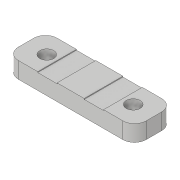
# Autodesk Inventor part: 8 peristaltic pump clamp 0.2mm
Saved by Autodesk Inventor 2020 (Build 240168000, 168)
## iProperties
Created: 2018-08-21
Part Number: 8 peristaltic pump clamp 0.2mm
Material: Generic
Document SubType Name: Modeling
Designer: mrbeh
Density: 1 g/cm^3
Appearance: Default
Author: mrbeh
Autodesk Inventor part; units mm, degrees
ref_plane "YZ Plane" through (0, 0, 0) normal (1, 0, 0) x (0, 1, 0)
ref_plane "XZ Plane" through (0, 0, 0) normal (0, 1, 0) x (-1, 0, 0)
sketch "Sketch1" plane through (0, 0, 0) normal (0, 1, 0) x (-1, 0, 0)
  line L0 (0, 0) -> (33, 0)
  line L1 (33, 0) -> (33, -10)
  line L2 (33, -10) -> (0, -10)
  line L3 (0, -10) -> (0, 0)
  dimension "d0" = 33
  dimension "d1" = 10
  constraints: 8 end point, 2 parallel, 1 horizontal, 1 perpendicular
  measures "d0" distance of L1.end L2.end
  measures "d1" distance of L0.end L1.end
extrude "Extrusion1" add sketch "Sketch1" along normal blind 4
sketch "Sketch2" plane through (0, 4, 0) normal (0, 1, 0) x (1, 0, 0)
  circle A0 centre (-5.343, 5) radius 1.8
  point P0 (0, 0)
  dimension "d9" = 3.6
  constraints: 1 centre point
  measures "d9" diameter of A0
extrude "Extrusion2" cut sketch "Sketch2" against normal blind 4
ref_plane "Work Plane1" through (-16.5, 0, 0) normal (1, 0, 0) x (0, 0, -1)
mirror "Mirror1" about plane through (-16.5, 0, 0) normal (1, 0, 0) of "Extrusion2"
fillet "Fillet1" radius 3 4 edges at (-33, 2, 0) (-33, 2, -10) (0, 2, 0) (0, 2, -10)
sketch "Sketch3" plane through (0, 4, 0) normal (0, 1, 0) x (1, 0, 0)
  line L0 (-30, 0) -> (-3, 0) projected
  line L1 (-30, 10) -> (-3, 10) projected
  line L2 (-20, 0) -> (-13, 0)
  line L3 (-13, 0) -> (-13, 10)
  line L4 (-13, 10) -> (-20, 10)
  line L5 (-20, 10) -> (-20, 0)
  point P0 (0, 0)
  dimension "d10" = 7
  dimension "d11" = 10
  constraints: 8 end point, 2 parallel, 1 horizontal, 1 perpendicular, 1 point on line
  measures "d10" distance of L4.end L3.end
  measures "d11" distance of L3.end L2.end
extrude "Extrusion3" add sketch "Sketch3" along normal blind 0.2
sketch "Sketch4" plane through (0, 4, 0) normal (0, 1, 0) x (1, 0, 0)
  line L0 (-3, 0) -> (-8, 0)
  line L1 (-8, 0) -> (-8, 10)
  line L2 (-8, 10) -> (-3, 10)
  line L3 (0, 7) -> (0, 3)
  arc A0 (-3, 0) -> (0, 3) centre (-3, 3) ccw
  arc A1 (0, 7) -> (-3, 10) centre (-3, 7) ccw
  circle A2 centre (-5.343, 5) radius 1.8 projected
  circle A3 centre (-5.343, 5) radius 1.8
  point P0 (0, 0)
  point P1 (0, 10)
  dimension "d14" = 8
  dimension "d15" = 10
  dimension "d16" = 3
  constraints: 8 end point, 4 point on circle, 4 point on line, 4 tangent, 3 centre point, 2 parallel, 1 coincident, 1 equal radius, 1 horizontal, 1 perpendicular
  measures "d14" distance of L1.end point (0, 10)
  measures "d15" distance of L0.end L1.end
  measures "d16" radius of A0
extrude "Extrusion4" add sketch "Sketch4" along normal blind 0.2
mirror "Mirror2" about plane through (-16.5, 0, 0) normal (1, 0, 0) of "Extrusion4"
sketch "Sketch5" plane through (0, 0, 0) normal (0, -1, 0) x (1, 0, 0)
  line L0 (-24.4942, -3.2042) -> (-8.1968, -3.2042) construction
  line L1 (-8.1968, -3.2042) -> (-8.1968, -6.8489) construction
  line L2 (-8.1968, -6.8489) -> (-24.4942, -6.8489) construction
  line L3 (-24.4942, -6.8489) -> (-24.4942, -3.2042) construction
  spline S0 degree 2 poles (-22.0607, -5.028) (-22.0607, -5.9696) (-22.6081, -6.8517) (-23.1782, -6.8517) knots 0 0 0 1 2 2 2
  spline S1 degree 2 poles (-23.1782, -6.8517) (-23.7568, -6.8517) (-24.2985, -5.9526) (-24.2985, -5.0308) knots 0 0 0 1 2 2 2
  spline S2 degree 2 poles (-24.2985, -5.0308) (-24.2985, -4.0835) (-23.7511, -3.2071) (-23.1782, -3.2071) knots 0 0 0 1 2 2 2
  spline S3 degree 2 poles (-23.1782, -3.2071) (-22.6024, -3.2071) (-22.0607, -4.1147) (-22.0607, -5.028) knots 0 0 0 1 2 2 2
  spline S4 degree 2 poles (-22.662, -6.0944) (-22.5939, -5.9214) (-22.5372, -5.3882) (-22.5372, -5.028) knots 0 0 0 1 2 2 2
  spline S5 degree 2 poles (-22.5372, -5.028) (-22.5372, -4.6678) (-22.5939, -4.1374) (-22.6648, -3.9587) knots 0 0 0 1 2 2 2
  spline S6 degree 2 poles (-22.6648, -3.9587) (-22.7357, -3.78) (-22.9825, -3.5957) (-23.1782, -3.5957) knots 0 0 0 1 2 2 2
  spline S7 degree 2 poles (-23.1782, -3.5957) (-23.3739, -3.5957) (-23.6263, -3.78) (-23.7, -3.9644) knots 0 0 0 1 2 2 2
  spline S8 degree 2 poles (-23.7, -3.9644) (-23.7709, -4.1431) (-23.822, -4.6876) (-23.822, -5.0308) knots 0 0 0 1 2 2 2
  spline S9 degree 2 poles (-23.822, -5.0308) (-23.822, -5.3995) (-23.7766, -5.8931) (-23.7029, -6.0859) knots 0 0 0 1 2 2 2
  spline S10 degree 2 poles (-23.7029, -6.0859) (-23.6348, -6.2675) (-23.3824, -6.4632) (-23.1782, -6.4632) knots 0 0 0 1 2 2 2
  spline S11 degree 2 poles (-23.1782, -6.4632) (-22.9853, -6.4632) (-22.7329, -6.2788) (-22.662, -6.0944) knots 0 0 0 1 2 2 2
  line L4 (-20.8609, -6.778) -> (-21.4225, -6.778)
  line L5 (-21.4225, -6.778) -> (-21.4225, -6.1086)
  line L6 (-21.4225, -6.1086) -> (-20.8609, -6.1086)
  line L7 (-20.8609, -6.1086) -> (-20.8609, -6.778)
  line L8 (-17.9962, -6.778) -> (-20.1547, -6.778)
  line L9 (-20.1547, -6.778) -> (-20.1547, -6.2816)
  spline S12 degree 2 poles (-20.1547, -6.2816) (-19.9221, -6.0632) (-19.508, -5.6576) (-19.3094, -5.4393) knots 0 0 0 1 2 2 2
  spline S13 degree 2 poles (-19.3094, -5.4393) (-18.9095, -4.9996) (-18.6174, -4.4721) (-18.6174, -4.1913) knots 0 0 0 1 2 2 2
  spline S14 degree 2 poles (-18.6174, -4.1913) (-18.6174, -4.0438) (-18.7081, -3.8226) (-18.7904, -3.7517) knots 0 0 0 1 2 2 2
  spline S15 degree 2 poles (-18.7904, -3.7517) (-18.8727, -3.6807) (-19.0882, -3.6098) (-19.2187, -3.6098) knots 0 0 0 1 2 2 2
  spline S16 degree 2 poles (-19.2187, -3.6098) (-19.3435, -3.6098) (-19.5987, -3.6722) (-19.715, -3.7205) knots 0 0 0 1 2 2 2
  spline S17 degree 2 poles (-19.715, -3.7205) (-19.8143, -3.7602) (-19.9987, -3.8736) (-20.0554, -3.9133) knots 0 0 0 1 2 2 2
  line L10 (-20.0554, -3.9133) -> (-20.0809, -3.9133)
  line L11 (-20.0809, -3.9133) -> (-20.0809, -3.4141)
  spline S18 degree 2 poles (-20.0809, -3.4141) (-19.9363, -3.3432) (-19.4172, -3.2042) (-19.1846, -3.2042) knots 0 0 0 1 2 2 2
  spline S19 degree 2 poles (-19.1846, -3.2042) (-18.694, -3.2042) (-18.1409, -3.7233) (-18.1409, -4.1658) knots 0 0 0 1 2 2 2
  spline S20 degree 2 poles (-18.1409, -4.1658) (-18.1409, -4.3728) (-18.2373, -4.7188) (-18.3224, -4.8663) knots 0 0 0 1 2 2 2
  spline S21 degree 2 poles (-18.3224, -4.8663) (-18.4075, -5.0195) (-18.6543, -5.3201) (-18.7904, -5.4648) knots 0 0 0 1 2 2 2
  spline S22 degree 2 poles (-18.7904, -5.4648) (-19.0116, -5.7059) (-19.5534, -6.2221) (-19.715, -6.3724) knots 0 0 0 1 2 2 2
  line L12 (-19.715, -6.3724) -> (-17.9962, -6.3724)
  line L13 (-17.9962, -6.3724) -> (-17.9962, -6.778)
  line L14 (-12.9816, -6.778) -> (-12.9816, -5.2577)
  spline S23 degree 2 poles (-12.9816, -5.2577) (-12.9816, -5.0762) (-13.01, -4.7671) (-13.0554, -4.682) knots 0 0 0 1 2 2 2
  spline S24 degree 2 poles (-13.0554, -4.682) (-13.1008, -4.5884) (-13.2738, -4.4976) (-13.4241, -4.4976) knots 0 0 0 1 2 2 2
  spline S25 degree 2 poles (-13.4241, -4.4976) (-13.5603, -4.4976) (-13.8722, -4.6649) (-14.0368, -4.8238) knots 0 0 0 1 2 2 2
  spline S26 degree 2 poles (-14.0368, -4.8238) (-14.0339, -4.8635) (-14.0282, -4.9741) (-14.0282, -5.0478) knots 0 0 0 1 2 2 2
  line L15 (-14.0282, -5.0478) -> (-14.0282, -6.778)
  line L16 (-14.0282, -6.778) -> (-14.4707, -6.778)
  line L17 (-14.4707, -6.778) -> (-14.4707, -5.2577)
  spline S27 degree 2 poles (-14.4707, -5.2577) (-14.4707, -5.0762) (-14.4991, -4.7671) (-14.5444, -4.682) knots 0 0 0 1 2 2 2
  spline S28 degree 2 poles (-14.5444, -4.682) (-14.5898, -4.5884) (-14.7628, -4.4976) (-14.9132, -4.4976) knots 0 0 0 1 2 2 2
  spline S29 degree 2 poles (-14.9132, -4.4976) (-15.055, -4.4976) (-15.3698, -4.6763) (-15.5173, -4.8153) knots 0 0 0 1 2 2 2
  line L18 (-15.5173, -4.8153) -> (-15.5173, -6.778)
  line L19 (-15.5173, -6.778) -> (-15.9598, -6.778)
  line L20 (-15.9598, -6.778) -> (-15.9598, -4.1516)
  line L21 (-15.9598, -4.1516) -> (-15.5173, -4.1516)
  line L22 (-15.5173, -4.1516) -> (-15.5173, -4.4409)
  spline S30 degree 2 poles (-15.5173, -4.4409) (-15.3443, -4.2679) (-15.0039, -4.0778) (-14.7997, -4.0778) knots 0 0 0 1 2 2 2
  spline S31 degree 2 poles (-14.7997, -4.0778) (-14.5671, -4.0778) (-14.2069, -4.2906) (-14.1133, -4.5316) knots 0 0 0 1 2 2 2
  spline S32 degree 2 poles (-14.1133, -4.5316) (-13.912, -4.3076) (-13.5319, -4.0778) (-13.3107, -4.0778) knots 0 0 0 1 2 2 2
  spline S33 degree 2 poles (-13.3107, -4.0778) (-13.1405, -4.0778) (-12.8625, -4.1828) (-12.7604, -4.3019) knots 0 0 0 1 2 2 2
  spline S34 degree 2 poles (-12.7604, -4.3019) (-12.6555, -4.421) (-12.5392, -4.7784) (-12.5392, -5.0478) knots 0 0 0 1 2 2 2
  line L23 (-12.5392, -5.0478) -> (-12.5392, -6.778)
  line L24 (-12.5392, -6.778) -> (-12.9816, -6.778)
  line L25 (-8.9399, -6.778) -> (-8.9399, -5.2577)
  spline S35 degree 2 poles (-8.9399, -5.2577) (-8.9399, -5.0762) (-8.9683, -4.7671) (-9.0137, -4.682) knots 0 0 0 1 2 2 2
  spline S36 degree 2 poles (-9.0137, -4.682) (-9.059, -4.5884) (-9.2321, -4.4976) (-9.3824, -4.4976) knots 0 0 0 1 2 2 2
  spline S37 degree 2 poles (-9.3824, -4.4976) (-9.5185, -4.4976) (-9.8305, -4.6649) (-9.995, -4.8238) knots 0 0 0 1 2 2 2
  spline S38 degree 2 poles (-9.995, -4.8238) (-9.9922, -4.8635) (-9.9865, -4.9741) (-9.9865, -5.0478) knots 0 0 0 1 2 2 2
  line L26 (-9.9865, -5.0478) -> (-9.9865, -6.778)
  line L27 (-9.9865, -6.778) -> (-10.429, -6.778)
  line L28 (-10.429, -6.778) -> (-10.429, -5.2577)
  spline S39 degree 2 poles (-10.429, -5.2577) (-10.429, -5.0762) (-10.4573, -4.7671) (-10.5027, -4.682) knots 0 0 0 1 2 2 2
  spline S40 degree 2 poles (-10.5027, -4.682) (-10.5481, -4.5884) (-10.7211, -4.4976) (-10.8714, -4.4976) knots 0 0 0 1 2 2 2
  spline S41 degree 2 poles (-10.8714, -4.4976) (-11.0133, -4.4976) (-11.3281, -4.6763) (-11.4756, -4.8153) knots 0 0 0 1 2 2 2
  line L29 (-11.4756, -4.8153) -> (-11.4756, -6.778)
  line L30 (-11.4756, -6.778) -> (-11.918, -6.778)
  line L31 (-11.918, -6.778) -> (-11.918, -4.1516)
  line L32 (-11.918, -4.1516) -> (-11.4756, -4.1516)
  line L33 (-11.4756, -4.1516) -> (-11.4756, -4.4409)
  spline S42 degree 2 poles (-11.4756, -4.4409) (-11.3026, -4.2679) (-10.9622, -4.0778) (-10.758, -4.0778) knots 0 0 0 1 2 2 2
  spline S43 degree 2 poles (-10.758, -4.0778) (-10.5254, -4.0778) (-10.1652, -4.2906) (-10.0716, -4.5316) knots 0 0 0 1 2 2 2
  spline S44 degree 2 poles (-10.0716, -4.5316) (-9.8702, -4.3076) (-9.4902, -4.0778) (-9.2689, -4.0778) knots 0 0 0 1 2 2 2
  spline S45 degree 2 poles (-9.2689, -4.0778) (-9.0987, -4.0778) (-8.8208, -4.1828) (-8.7187, -4.3019) knots 0 0 0 1 2 2 2
  spline S46 degree 2 poles (-8.7187, -4.3019) (-8.6137, -4.421) (-8.4974, -4.7784) (-8.4974, -5.0478) knots 0 0 0 1 2 2 2
  line L34 (-8.4974, -5.0478) -> (-8.4974, -6.778)
  line L35 (-8.4974, -6.778) -> (-8.9399, -6.778)
  point P0 (0, 0)
  constraints: 2 other
extrude "Extrusion5" add sketch "Sketch5" along normal blind 0.5
body "Solid1"
